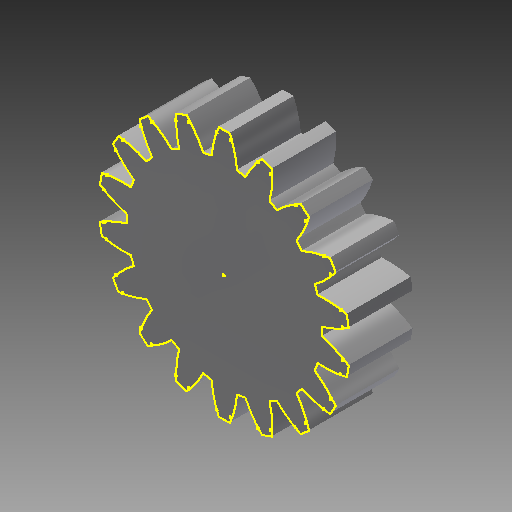
# Autodesk Inventor part: Цилиндрическое зубчатое зацепление1
Saved by Autodesk Inventor 2019 (Build 230136000, 136)
## iProperties
Created: 2020-02-27
Part Number: Цилиндрическое зубчатое зацепление1
Material: Steel
Document SubType Name: Modeling
Designer: Петров Иван
Categories: <?xml version="1.0" encoding="UTF-16"?> <MemberInstance><Categories><FamilyTemplate><FamilyTemplateParameter ValueType="xs:double" Id="1" ObjectReferenceKey="da_z" ObjectType="kUserParameterObject"/><FamilyTemplateParameter ValueType="xs:double" Id="2" ObjectReferenceKey="da_b" ObjectType="kUserParameterObject"/><FamilyTemplateParameter ValueType="xs:double" Id="3" ObjectReferenceKey="da_beta" ObjectType="kUserParameterObject"/><FamilyTemplateParameter ValueType="xs:double" Id="4" ObjectReferenceKey="da_da" ObjectType="kUserParameterObject"/><FamilyTemplateParameter ValueType="xs:double" Id="5" ObjectReferenceKey="da_aw" ObjectType="kUserParameterObject"/><FamilyTemplateParameter ValueType="xs:string" Id="6" ObjectReferenceKey="EAIAABAAAACIAQAAAAAAAIAAAAAAAAAA" ObjectType="83910656" SubObjectId="SurfaceGeometry"/></FamilyTemplate><ParamToTemplateMap><ParamToTemplate CategoryParameter="//CategoryParameter[@InternalName='046C89C9-8512-4d59-83FE-43B91F4F132A']" TemplateParameter="1"/><ParamToTemplate CategoryParameter="//CategoryParameter[@InternalName='2552DF32-E462-4b46-AEBF-C6C7768E72AC']" TemplateParameter="2"/><ParamToTemplate CategoryParameter="//CategoryParameter[@InternalName='C9EE641D-15FC-4fae-A226-E94C4372FDD7']" TemplateParameter="3"/><ParamToTemplate><ParamToTemplate CategoryParameter="//CategoryParameter[@InternalName='00B6519A-459B-49c7-AD84-2E56D39A5744']" ConstantValue="0.000000"/></ParamToTemplate><ParamToTemplate><ParamToTemplate CategoryParameter="//CategoryParameter[@InternalName='04B31F0E-C7A6-4894-AA32-9629BEFACF47']" ConstantValue="1.000000"/></ParamToTemplate><ParamToTemplate><ParamToTemplate CategoryParameter="//CategoryParameter[@InternalName='43CBEC2E-7847-49e7-A936-2F7889FCB2D9']" ConstantValue="0.250000"/></ParamToTemplate><ParamToTemplate><ParamToTemplate CategoryParameter="//CategoryParameter[@InternalName='B1EFC894-105D-4ebd-86BF-FA20ED196853']" ConstantValue="0.350000"/></ParamToTemplate><ParamToTemplate><ParamToTemplate CategoryParameter="//CategoryParameter[@InternalName='51175063-3D10-4879-93E8-6246FE8B403D']" ConstantValue="2060000000.000000"/></ParamToTemplate><ParamToTemplate><ParamToTemplate CategoryParameter="//CategoryParameter[@InternalName='A3A52E27-4454-46a9-B0BD-C932399B70AF']" ConstantValue="0.300000"/></ParamToTemplate><ParamToTemplate><ParamToTemplate CategoryParameter="//CategoryParameter[@InternalName='91B76062-C214-41d9-B1B9-14D2AB99603D']" ConstantValue="0.137500"/></ParamToTemplate><ParamToTemplate><ParamToTemplate CategoryParameter="//CategoryParameter[@InternalName='374E806E-8B8A-4dda-A9AA-1039D6500AD2']" ConstantValue="7.272727"/></ParamToTemplate><ParamToTemplate><ParamToTemplate CategoryParameter="//CategoryParameter[@InternalName='2D373A89-B862-43d6-8D0B-0CBF12AB9F6C']" ConstantValue="0.523599"/></ParamToTemplate><ParamToTemplate CategoryParameter="//CategoryParameter[@InternalName='37777632-D6A2-4fac-9D53-DB8ACD95C989']" TemplateParameter="4"/><ParamToTemplate CategoryParameter="//CategoryParameter[@InternalName='FD1017F1-B727-4f7e-9707-0F86F1FF9423']" TemplateParameter="5"/><ParamToTemplate><ParamToTemplate CategoryParameter="//CategoryParameter[@InternalName='9E1B4470-B2D3-4ff1-B813-535BB4CDF51A']" ConstantValue="3520000.000000"/></ParamToTemplate><ParamToTemplate><ParamToTemplate CategoryParameter="//CategoryParameter[@InternalName='F8452263-BFF6-458c-9FB1-07C4B99E95CD']" ConstantValue="11400000.000000"/></ParamToTemplate><ParamToTemplate><ParamToTemplate CategoryParameter="//CategoryParameter[@InternalName='3E3BB259-FD49-497f-8171-6EBC954A3479']" ConstantValue="2.000000"/></ParamToTemplate><ParamToTemplate CategoryParameter="//CategoryParameter[@InternalName='27C3BAF2-7550-4e4b-AE2C-0DB134B7D9B7']" TemplateParameter="6"/></ParamToTemplateMap><Category DisplayName="Gear" InternalName="DC85795E-93AB-48d5-8EEE-5A27447B64BD" Mnemonic="Gear"><CategoryParameter DisplayName="z" InternalName="046C89C9-8512-4d59-83FE-43B91F4F132A" Mnemonic="z"/><CategoryParameter DisplayName="b" InternalName="2552DF32-E462-4b46-AEBF-C6C7768E72AC" Mnemonic="b"/><CategoryParameter DisplayName="||b|" InternalName="C9EE641D-15FC-4fae-A226-E94C4372FDD7" Mnemonic="beta"/><CategoryParameter DisplayName="x" InternalName="00B6519A-459B-49c7-AD84-2E56D39A5744" Mnemonic="x"/><CategoryParameter DisplayName="a*" InternalName="04B31F0E-C7A6-4894-AA32-9629BEFACF47" Mnemonic="a"/><CategoryParameter DisplayName="c*" InternalName="43CBEC2E-7847-49e7-A936-2F7889FCB2D9" Mnemonic="c"/><CategoryParameter DisplayName="r|.f|*" InternalName="B1EFC894-105D-4ebd-86BF-FA20ED196853" Mnemonic="rf"/><CategoryParameter DisplayName="E" InternalName="51175063-3D10-4879-93E8-6246FE8B403D" Mnemonic="E"/><CategoryParameter DisplayName="||m|" InternalName="A3A52E27-4454-46a9-B0BD-C932399B70AF" Mnemonic="mi"/><Category DisplayName="SpurGear" InternalName="26C5A22E-A91E-4dfd-A3B3-23CCAFAE1764" Mnemonic="SpurGear"><CategoryParameter DisplayName="m" InternalName="91B76062-C214-41d9-B1B9-14D2AB99603D" Mnemonic="m"/><CategoryParameter DisplayName="P" InternalName="374E806E-8B8A-4dda-A9AA-1039D6500AD2" Mnemonic="PP"/><CategoryParameter DisplayName="||a|" InternalName="2D373A89-B862-43d6-8D0B-0CBF12AB9F6C" Mnemonic="alpha"/><CategoryParameter DisplayName="d|.a|" InternalName="37777632-D6A2-4fac-9D53-DB8ACD95C989" Mnemonic="da"/><CategoryParameter DisplayName="a|.w|" InternalName="FD1017F1-B727-4f7e-9707-0F86F1FF9423" Mnemonic="aw"/><CategoryParameter DisplayName="||s||.Flim|" InternalName="9E1B4470-B2D3-4ff1-B813-535BB4CDF51A" Mnemonic="sFlim"/><CategoryParameter DisplayName="||s||.Hlim|" InternalName="F8452263-BFF6-458c-9FB1-07C4B99E95CD" Mnemonic="sHlim"/><CategoryParameter DisplayName="тип" InternalName="3E3BB259-FD49-497f-8171-6EBC954A3479" Mnemonic="type"/><CategoryParameter DisplayName="PitchDiameter" InternalName="27C3BAF2-7550-4e4b-AE2C-0DB134B7D9B7" Mnemonic="IDS_PITCHDIAM"/></Category></Category></Categories></MemberInstance>
Density: 1 g/cm^3
Appearance: Steel
CustomPartVersion: 1
Author: Петров Иван
Autodesk Inventor part; units mm, degrees
sketch "Sketch1" plane through (0, 0, 0) normal (0, 0, 1) x (1, 0, 0)
  circle A0 centre (0, 0) radius 13.6591
  dimension "d0" = 27.3182
  constraints: 1 centre point
  measures "d0" diameter of A0
extrude "Extrusion1" add sketch "Sketch1" along normal blind 7
ref_plane "Work Plane2" through (0, 0, 3.5) normal (0, 0, 1) x (1, 0, 0)
sketch "Sketch2" plane through (0, 0, 0) normal (0, 0, -1) x (-1, 0, 0)
  circle A0 centre (0, 0) radius 13.6591 projected
  circle A1 centre (0, 0) radius 12
  dimension "d3" = 24
  constraints: 1 centre point, 1 coincident
  measures "d3" diameter of A1
surface extrude "Средний диаметр" sketch "Sketch2" against normal through all shown no curves A1
ref_plane "Work Plane8" through (0, 0, 0) normal (0.9848078, 0.1736482, 0) x (0, 0, 1)
ref_plane "Work Plane9" through (0, 0, 0) normal (1, 0, 0) x (0, 1, 0)
spur gear teeth "Цилиндрическое зубчатое зацепление" teeth 18 pitch diameter 24.75 tip diameter 27.3182 root diameter 21.3125 face width 7 start plane through (0, 0, 0) normal (0, 0, -1) x (-1, 0, 0)
sketch "Эскиз3" plane through (0, 0, 7) normal (0, 0, 1) x (1, 0, 0)
  arc A0 (-5.2271, 12.6194) -> (-4.9205, 9.4522) centre (5.1709, 12.0276) ccw projected
  arc A1 (-4.9205, 9.4522) -> (-5.7256, 8.9874) centre (0, 0) ccw projected
  arc A2 (-5.7256, 8.9874) -> (-8.3151, 10.8365) centre (-13.0016, 1.5357) ccw projected
  arc A3 (-8.3151, 10.8365) -> (-9.228, 10.0706) centre (0, 0) ccw projected
  arc A4 (-9.228, 10.0706) -> (-7.8566, 7.1993) centre (0.7454, 13.0708) ccw projected
  arc A5 (-7.8566, 7.1993) -> (-8.4542, 6.4871) centre (0, 0) ccw projected
  arc A6 (-8.4542, 6.4871) -> (-11.52, 7.339) centre (-12.7428, -3.0038) ccw projected
  arc A7 (-11.52, 7.339) -> (-12.1158, 6.3071) centre (0, 0) ccw projected
  arc A8 (-12.1158, 6.3071) -> (-9.8451, 4.078) centre (-3.77, 12.5374) ccw projected
  arc A9 (-9.8451, 4.078) -> (-10.163, 3.2044) centre (0, 0) ccw projected
  arc A10 (-10.163, 3.2044) -> (-13.3353, 2.9564) centre (-10.9469, -7.1809) ccw projected
  arc A11 (-13.3353, 2.9564) -> (-13.5423, 1.7829) centre (0, 0) ccw projected
  arc A12 (-13.5423, 1.7829) -> (-10.6461, 0.4648) centre (-7.8307, 10.4919) ccw projected
  arc A13 (-10.6461, 0.4648) -> (-10.6461, -0.4648) centre (0, 0) ccw projected
  arc A14 (-10.6461, -0.4648) -> (-13.5423, -1.7829) centre (-7.8307, -10.4919) ccw projected
  arc A15 (-13.5423, -1.7829) -> (-13.3353, -2.9564) centre (0, 0) ccw projected
  arc A16 (-13.3353, -2.9564) -> (-10.163, -3.2044) centre (-10.9469, 7.1809) ccw projected
  arc A17 (-10.163, -3.2044) -> (-9.8451, -4.078) centre (0, 0) ccw projected
  arc A18 (-9.8451, -4.078) -> (-12.1158, -6.3071) centre (-3.77, -12.5374) ccw projected
  arc A19 (-12.1158, -6.3071) -> (-11.52, -7.339) centre (0, 0) ccw projected
  arc A20 (-11.52, -7.339) -> (-8.4542, -6.4871) centre (-12.7428, 3.0038) ccw projected
  arc A21 (-8.4542, -6.4871) -> (-7.8566, -7.1993) centre (0, 0) ccw projected
  arc A22 (-7.8566, -7.1993) -> (-9.228, -10.0706) centre (0.7454, -13.0708) ccw projected
  arc A23 (-9.228, -10.0706) -> (-8.3151, -10.8365) centre (0, 0) ccw projected
  arc A24 (-8.3151, -10.8365) -> (-5.7256, -8.9874) centre (-13.0016, -1.5357) ccw projected
  arc A25 (-5.7256, -8.9874) -> (-4.9205, -9.4522) centre (0, 0) ccw projected
  arc A26 (-4.9205, -9.4522) -> (-5.2271, -12.6194) centre (5.1709, -12.0276) ccw projected
  arc A27 (-5.2271, -12.6194) -> (-4.1074, -13.0269) centre (0, 0) ccw projected
  arc A28 (-4.1074, -13.0269) -> (-2.3064, -10.4037) centre (-11.6923, -5.8899) ccw projected
  arc A29 (-2.3064, -10.4037) -> (-1.3909, -10.5651) centre (0, 0) ccw projected
  arc A30 (-1.3909, -10.5651) -> (-0.5958, -13.6461) centre (8.9727, -9.5337) ccw projected
  arc A31 (-0.5958, -13.6461) -> (0.5958, -13.6461) centre (0, 0) ccw projected
  arc A32 (0.5958, -13.6461) -> (1.3909, -10.5651) centre (-8.9727, -9.5337) ccw projected
  arc A33 (1.3909, -10.5651) -> (2.3064, -10.4037) centre (0, 0) ccw projected
  arc A34 (2.3064, -10.4037) -> (4.1074, -13.0269) centre (11.6923, -5.8899) ccw projected
  arc A35 (4.1074, -13.0269) -> (5.2271, -12.6194) centre (0, 0) ccw projected
  arc A36 (5.2271, -12.6194) -> (4.9205, -9.4522) centre (-5.1709, -12.0276) ccw projected
  arc A37 (4.9205, -9.4522) -> (5.7256, -8.9874) centre (0, 0) ccw projected
  arc A38 (5.7256, -8.9874) -> (8.3151, -10.8365) centre (13.0016, -1.5357) ccw projected
  arc A39 (8.3151, -10.8365) -> (9.228, -10.0706) centre (0, 0) ccw projected
  arc A40 (9.228, -10.0706) -> (7.8566, -7.1993) centre (-0.7454, -13.0708) ccw projected
  arc A41 (7.8566, -7.1993) -> (8.4542, -6.4871) centre (0, 0) ccw projected
  arc A42 (8.4542, -6.4871) -> (11.52, -7.339) centre (12.7428, 3.0038) ccw projected
  arc A43 (11.52, -7.339) -> (12.1158, -6.3071) centre (0, 0) ccw projected
  arc A44 (12.1158, -6.3071) -> (9.8451, -4.078) centre (3.77, -12.5374) ccw projected
  arc A45 (9.8451, -4.078) -> (10.163, -3.2044) centre (0, 0) ccw projected
  arc A46 (10.163, -3.2044) -> (13.3353, -2.9564) centre (10.9469, 7.1809) ccw projected
  arc A47 (13.3353, -2.9564) -> (13.5423, -1.7829) centre (0, 0) ccw projected
  arc A48 (13.5423, -1.7829) -> (10.6461, -0.4648) centre (7.8307, -10.4919) ccw projected
  arc A49 (10.6461, -0.4648) -> (10.6461, 0.4648) centre (0, 0) ccw projected
  arc A50 (10.6461, 0.4648) -> (13.5423, 1.7829) centre (7.8307, 10.4919) ccw projected
  arc A51 (13.5423, 1.7829) -> (13.3353, 2.9564) centre (0, 0) ccw projected
  arc A52 (13.3353, 2.9564) -> (10.163, 3.2044) centre (10.9469, -7.1809) ccw projected
  arc A53 (10.163, 3.2044) -> (9.8451, 4.078) centre (0, 0) ccw projected
  arc A54 (9.8451, 4.078) -> (12.1158, 6.3071) centre (3.77, 12.5374) ccw projected
  arc A55 (12.1158, 6.3071) -> (11.52, 7.339) centre (0, 0) ccw projected
  arc A56 (11.52, 7.339) -> (8.4542, 6.4871) centre (12.7428, -3.0038) ccw projected
  arc A57 (8.4542, 6.4871) -> (7.8566, 7.1993) centre (0, 0) ccw projected
  arc A58 (7.8566, 7.1993) -> (9.228, 10.0706) centre (-0.7454, 13.0708) ccw projected
  arc A59 (9.228, 10.0706) -> (8.3151, 10.8365) centre (0, 0) ccw projected
  arc A60 (8.3151, 10.8365) -> (5.7256, 8.9874) centre (13.0016, 1.5357) ccw projected
  arc A61 (5.7256, 8.9874) -> (4.9205, 9.4522) centre (0, 0) ccw projected
  arc A62 (4.9205, 9.4522) -> (5.2271, 12.6194) centre (-5.1709, 12.0276) ccw projected
  arc A63 (5.2271, 12.6194) -> (4.1074, 13.0269) centre (0, 0) ccw projected
  arc A64 (4.1074, 13.0269) -> (2.3064, 10.4037) centre (11.6923, 5.8899) ccw projected
  arc A65 (2.3064, 10.4037) -> (1.3909, 10.5651) centre (0, 0) ccw projected
  arc A66 (1.3909, 10.5651) -> (0.5958, 13.6461) centre (-8.9727, 9.5337) ccw projected
  arc A67 (0.5958, 13.6461) -> (-0.5958, 13.6461) centre (0, 0) ccw projected
  arc A68 (-0.5958, 13.6461) -> (-1.3909, 10.5651) centre (8.9727, 9.5337) ccw projected
  arc A69 (-1.3909, 10.5651) -> (-2.3064, 10.4037) centre (0, 0) ccw projected
  arc A70 (-2.3064, 10.4037) -> (-4.1074, 13.0269) centre (-11.6923, 5.8899) ccw projected
  arc A71 (-4.1074, 13.0269) -> (-5.2271, 12.6194) centre (0, 0) ccw projected
equation "\"d0\" = da_da"
equation "\"d1\" = da_b"
equation "\"d3\" = da_dw"
equation "\"da_da\" = 27.318247"
equation "\"da_b\" = 7"
equation "\"da_dw\" = 24"
body "Solid1"
body "Srf1"
